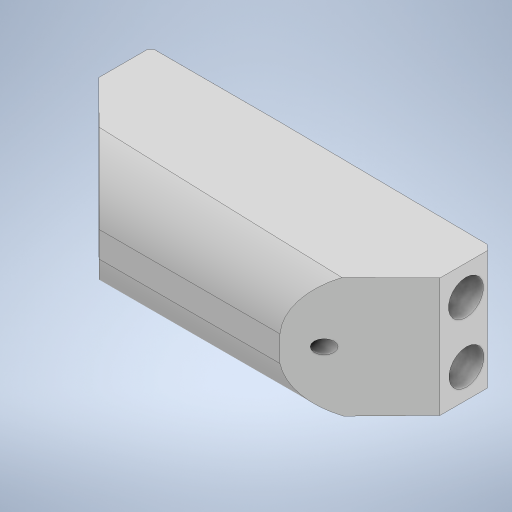
# Autodesk Inventor part: Mittelfinger middle
Saved by Autodesk Inventor 2024 (Build 280153000, 153)
## iProperties
Created: 2025-05-19
Part Number: Mittelfinger middle
Material: Generic
Document SubType Name: Modeling
Designer: Mehdi Charfeddine
Density: 1 g/cm^3
Appearance: Default
Author: Mehdi Charfeddine
Autodesk Inventor part; units mm, degrees
ref_plane "YZ Plane" through (0, 0, 0) normal (1, 0, 0) x (0, 1, 0)
ref_plane "XZ Plane" through (0, 0, 0) normal (0, 1, 0) x (-1, 0, 0)
ref_plane "XY Plane" through (0, 0, 0) normal (0, 0, 1) x (1, 0, 0)
sketch "Sketch1" plane through (0, 0, 0) normal (1, 0, 0) x (0, 1, 0)
  line L0 (340.282, 0) -> (-10.8388, 0)
  line L1 (-10.8388, 0) -> (-25.5507, 15.2858)
  line L2 (-25.5507, 15.2858) -> (-25.5507, 217.175)
  line L3 (-25.5507, 217.175) -> (-38.993, 226.1376)
  line L4 (340.282, 0) -> (355.4347, 15.2858)
  line L5 (355.4347, 15.2858) -> (355.4347, 217.175)
  line L6 (355.4347, 217.175) -> (367.563, 217.175)
  arc A0 (355.4347, 217.175) -> (195.0461, 381.0987) centre (188.4409, 214.2093) ccw
  arc A1 (124.0848, 381.0987) -> (-25.5507, 217.175) centre (143.9158, 212.7381) ccw
  line L7 (195.0461, 381.0987) -> (124.0848, 381.0987)
  arc A2 (175.1634, 293.3237) -> (190.9337, 321.9969) centre (164.6697, 317.7686) ccw
  arc A3 (297.7202, 42.191) -> (295.1132, 116.2304) centre (249.3573, 77.5537) ccw
  arc A4 (35.0505, 112.9556) -> (31.2213, 44.0285) centre (76.6419, 76.075) ccw
  circle A5 centre (249.3573, 77.5537) radius 50
  circle A6 centre (76.6419, 76.075) radius 50
  circle A7 centre (164.6697, 317.7686) radius 20
  point P0 (0, 0)
  dimension "d0" = 100
  dimension "d1" = 100
  dimension "d2" = 40
  constraints: 16 end point, 10 point on circle, 8 centre point, 3 coincident, 2 horizontal, 2 perpendicular, 1 vertical
  measures "d0" diameter of A5
  measures "d1" diameter of A6
  measures "d2" diameter of A7
extrude "Extrusion1" add sketch "Sketch1" along normal mid plane 3700
sketch "Sketch2" plane through (0, 0, 0) normal (0, 0, 1) x (1, 0, 0)
  line L0 (-965.5809, 355.48) -> (-114.2964, 338.8136)
  line L1 (-114.2964, 338.8136) -> (-114.2964, -25.4428)
  line L2 (-114.2964, -25.4428) -> (-965.5809, -25.4428)
  line L3 (-965.5809, -25.4428) -> (-965.5809, 355.48)
  line L4 (66.842, 345.337) -> (66.842, -14.6982)
  line L5 (66.842, -14.6982) -> (790.3003, -8.0801)
  line L6 (790.3003, -8.0801) -> (790.3003, 337.3259)
  line L7 (790.3003, 337.3259) -> (66.842, 345.337)
  line L8 (953.6462, 335.5171) -> (952.4956, -5.9793)
  line L9 (952.4956, -5.9793) -> (1439.2474, -1.5266)
  line L10 (1439.2474, -1.5266) -> (1436.1794, 333.8533)
  line L11 (1436.1794, 333.8533) -> (1439.2234, 333.8811)
  line L12 (1439.2234, 333.8811) -> (953.6462, 335.5171)
  line L13 (953.6462, 335.5171) -> (952.4956, -5.9793)
  arc A0 (1575.7881, 200.0109) -> (1439.2234, 333.8811) centre (1440.4614, 198.5523) ccw
  arc A1 (1439.2474, -1.5266) -> (1575.7881, 129.0143) centre (1442.7286, 131.5108) ccw
  line L14 (1575.7881, 200.0109) -> (1575.7881, 129.0143)
  line L15 (-3435.0106, 1002.6799) -> (3280.5357, 1002.6799)
  line L16 (3280.5357, 1002.6799) -> (3280.5357, -1215.7591)
  line L17 (3280.5357, -1215.7591) -> (-3435.0106, -1215.7591)
  line L18 (-3435.0106, -1215.7591) -> (-3435.0106, 1002.6799)
  point P0 (0, 0)
  constraints: 38 end point, 6 perpendicular, 4 point on circle, 3 parallel, 3 vertical, 2 centre point, 1 horizontal, 1 tangent
extrude "Extrusion2" cut sketch "Sketch2" along normal mid plane 3700
sketch "Sketch3" plane through (0, 0, 0) normal (0, 1, 0) x (-1, 0, 0)
  line L0 (951.3287, 1.0445) -> (130.7941, 1.0445)
  line L1 (130.7941, 1.0445) -> (113.7889, 16.9983)
  line L2 (113.7889, 16.9983) -> (113.7889, 151.3461)
  line L3 (113.7889, 151.3461) -> (343.5511, 382.205)
  line L4 (343.5511, 382.205) -> (736.724, 382.205)
  line L5 (736.724, 382.205) -> (968.6848, 151.3461)
  line L6 (968.6848, 151.3461) -> (967.4264, 17.219)
  line L7 (967.4264, 17.219) -> (951.3287, 1.0445)
  line L8 (-295.326, 381.023) -> (-562.058, 381.023)
  line L9 (-562.058, 381.023) -> (-790.589, 151.4011)
  line L10 (-790.589, 151.4011) -> (-790.589, 16.1745)
  line L11 (-790.589, 16.1745) -> (-774.4619, 1.0445)
  line L12 (-774.4619, 1.0445) -> (-80.7583, 1.0445)
  line L13 (-80.7583, 1.0445) -> (-65.6576, 16.2172)
  line L14 (-65.6576, 16.2172) -> (-65.6576, 152.4456)
  line L15 (-65.6576, 152.4456) -> (-295.326, 381.023)
  line L16 (-952.2126, 153.4901) -> (-952.2126, 16.2172)
  line L17 (-952.2126, 16.2172) -> (-967.3132, 1.0445)
  line L18 (-967.3132, 1.0445) -> (-1428.6311, 1.0445)
  line L19 (-1428.6311, 1.0445) -> (-1574.2483, 158.5669)
  line L20 (-1574.2483, 158.5669) -> (-1575.0482, 186.0708)
  line L21 (-952.2126, 153.4901) -> (-1180.6664, 371.7672)
  line L22 (-1180.6664, 371.7672) -> (-1408.3189, 362.7531)
  arc A0 (-1408.3189, 362.7531) -> (-1575.0482, 186.0708) centre (-1396.965, 185.0292) ccw
  line L23 (1233.367, 649.2551) -> (-1898.5263, 649.2551)
  line L24 (-1898.5263, 649.2551) -> (-1898.5263, -608.2524)
  line L25 (-1898.5263, -608.2524) -> (1233.367, -608.2524)
  line L26 (1233.367, -608.2524) -> (1233.367, 649.2551)
  point P0 (0, 0)
  constraints: 54 end point, 7 parallel, 7 perpendicular, 4 point on line, 3 horizontal, 2 point on circle, 1 centre point, 1 vertical
extrude "Extrusion3" cut sketch "Sketch3" along normal mid plane 3700
sketch "Sketch4" plane through (-130.7941, -11.844, 1.0445) normal (0, 0, -1) x (-1, 0, 0)
  line L0 (1231.0766, 642.5401) -> (1231.0766, -266.4042)
  line L1 (1231.0766, -266.4042) -> (-106.4675, -266.4042)
  line L2 (-106.4675, -266.4042) -> (-106.4675, 748.6156)
  line L3 (-106.4675, 748.6156) -> (1231.0766, 748.6156)
  line L4 (1231.0766, 748.6156) -> (1231.0766, -266.4042)
  line L5 (-1006.2939, -298.7234) -> (-2002.0035, -298.7234)
  line L6 (-2002.0035, -298.7234) -> (-2002.0035, 789.1815)
  line L7 (-2002.0035, 789.1815) -> (-1006.2939, 789.1815)
  line L8 (-1006.2939, 789.1815) -> (-1006.2939, -298.7234)
  point P0 (-130.7941, 11.844)
  point P1 (1231.0766, 642.5401)
  constraints: 18 end point, 4 parallel, 2 horizontal, 2 perpendicular
extrude "Extrusion5" cut sketch "Sketch4" along normal mid plane 2000
move faces "Move2" translate (250, 0, 0) faces at (790.3003, 189.6162, 143.3251) (779.7413, 222.2007, 5.9975) (741.8383, 164.532, 200.3845)
sketch "Sketch5" plane through (429.845, 341.3173, 1.0445) normal (0, 0, -1) x (-1, 0, 0)
  circle A0 centre (-523.4536, -67.6305) radius 19.5608
  point P0 (429.845, -341.3173)
  constraints: 1 centre point
extrude "Extrusion6" cut sketch "Sketch5" against normal blind 5
body "Solid1"
